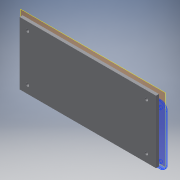
# Autodesk Inventor part: case_bot
Saved by Autodesk Inventor 2019 (Build 230136000, 136)
## iProperties
Created: 2020-04-18
Part Number: case_bot
Material: Generisch
Document SubType Name: Modeling
Designer: marc
Density: 1 g/cm^3
Appearance: Vorgabe
Author: marc
Autodesk Inventor part; units mm, degrees
ref_plane "YZ Plane" through (0, 0, 0) normal (1, 0, 0) x (0, 1, 0)
ref_plane "XZ Plane" through (0, 0, 0) normal (0, 1, 0) x (-1, 0, 0)
ref_plane "XY Plane" through (0, 0, 0) normal (0, 0, 1) x (1, 0, 0)
ref_plane "Arbeitsebene1" through (0, 0, 0) normal (0, 0, 1) x (1, 0, 0)
sketch "Skizze1" plane through (0, 0, 0) normal (0, 0, 1) x (1, 0, 0)
  circle A0 centre (-59.69, 23.2744) radius 1.6 projected
  circle A1 centre (59.69, 23.2744) radius 1.6 projected
  circle A2 centre (59.69, -23.7156) radius 1.6 projected
  circle A3 centre (-59.69, -23.7156) radius 1.6 projected
  circle A4 centre (-59.69, 23.2744) radius 3
  circle A5 centre (59.69, 23.2744) radius 3
  circle A6 centre (59.69, -23.7156) radius 3
  circle A7 centre (-59.69, -23.7156) radius 3
  point P0 (0, 0)
  dimension "d0" = 6
  dimension "d1" = 6
  dimension "d2" = 6
  dimension "d3" = 6
  constraints: 4 centre point, 4 coincident
  measures "d0" diameter of A4
  measures "d1" diameter of A7
  measures "d2" diameter of A5
  measures "d3" diameter of A6
extrude "Extrusion1" add sketch "Skizze1" along normal blind 3
ref_plane "Arbeitsebene2" through (0, 0, 0) normal (0, 0, 1) x (1, 0, 0)
sketch "Skizze2" plane through (0, 0, 0) normal (0, 0, 1) x (1, 0, 0)
  line L0 (-30.04, 15.6244) -> (-27.04, 15.6244)
  line L1 (-27.04, -19.3756) -> (-30.04, -19.3756)
  line L2 (-20.04, 0.6244) -> (-20.04, -4.3756)
  line L3 (-37.04, -4.3756) -> (-37.04, 0.6244)
  line L4 (-1.04, 9.6244) -> (3.96, 9.6244)
  line L5 (3.96, -8.3756) -> (-1.04, -8.3756)
  line L6 (10.96, 0.6244) -> (10.96, -4.3756)
  line L7 (-8.04, -4.3756) -> (-8.04, 0.6244)
  line L8 (40.96, -1.3756) -> (53.96, -1.3756)
  line L9 (53.96, -1.3756) -> (53.96, -4.3756)
  line L10 (53.96, -4.3756) -> (40.96, -4.3756)
  line L11 (40.96, -4.3756) -> (40.96, -1.3756)
  line L12 (-8.04, 0.6244) -> (-1.04, 0.6244)
  line L13 (3.96, 0.6244) -> (10.96, 0.6244)
  line L14 (3.96, 9.6244) -> (3.96, 0.6244)
  line L15 (3.96, -4.3756) -> (3.96, -8.3756)
  line L16 (10.96, -4.3756) -> (3.96, -4.3756)
  line L17 (-1.04, -4.3756) -> (-8.04, -4.3756)
  line L18 (-1.04, -8.3756) -> (-1.04, -4.3756)
  line L19 (-1.04, 0.6244) -> (-1.04, 9.6244)
  line L20 (-37.04, 0.6244) -> (-30.04, 0.6244)
  line L21 (-27.04, 0.6244) -> (-20.04, 0.6244)
  line L22 (-27.04, 15.6244) -> (-27.04, 0.6244)
  line L23 (-27.04, -4.3756) -> (-27.04, -19.3756)
  line L24 (-30.04, -19.3756) -> (-30.04, -4.3756)
  line L25 (-30.04, 0.6244) -> (-30.04, 15.6244)
  line L26 (-20.04, -4.3756) -> (-27.04, -4.3756)
  line L27 (-30.04, -4.3756) -> (-37.04, -4.3756)
  line L28 (-66.04, -24.3506) -> (-66.04, 23.2744) projected
  line L29 (-59.69, 29.6244) -> (59.69, 29.6244) projected
  point P0 (0, 0)
  dimension "d6" = 3
  dimension "d7" = 7
  dimension "d8" = 7
  dimension "d9" = 7
  dimension "d10" = 7
  dimension "d11" = 3
  dimension "d12" = 15
  dimension "d13" = 15
  dimension "d14" = 15
  dimension "d15" = 15
  dimension "d16" = 5
  dimension "d17" = 29
  dimension "d18" = 14
  dimension "d19" = 20
  dimension "d20" = 18
  dimension "d21" = 7
  dimension "d22" = 7
  dimension "d23" = 12
  dimension "d24" = 5
  dimension "d25" = 13
  dimension "d26" = 30
  dimension "d27" = 31
  constraints: 56 end point, 22 parallel, 9 perpendicular, 7 horizontal, 4 horizontal alignment, 2 vertical alignment
  measures "d6" distance of L8.end L9.end
  measures "d7" distance of L21.start L2.start
  measures "d8" distance of L3.end L20.end
  measures "d9" distance of L24.end L3.start
  measures "d10" distance of L2.end L23.start
  measures "d11" distance of L1.start L1.end
  measures "d12" distance of L0.end L21.start
  measures "d13" distance of L23.start L1.start
  measures "d14" distance of L20.end L0.start
  measures "d15" distance of L1.end L24.end
  measures "d16" distance of L2.start L2.end
  measures "d17" distance between parallel lines of L28 L3
  measures "d18" distance between parallel lines of L29 L0
  measures "d19" distance between parallel lines of L29 L4
  measures "d20" distance between parallel lines of L4 L5
  measures "d21" distance of L7.end L12.end
  measures "d22" distance of L13.start L6.start
  measures "d23" distance between parallel lines of L2 L7
  measures "d24" distance of L5.start L5.end
  measures "d25" distance of L8.start L8.end
  measures "d26" distance between parallel lines of L6 L11
  measures "d27" distance between parallel lines of L29 L8
extrude "Extrusion2" add sketch "Skizze2" along normal up to surface (3 mm away)
sketch "Skizze3" plane through (-8.04, 0.6244, 3) normal (0, 0, 1) x (1, 0, 0)
  line L0 (-59.65, 30.65) -> (77.33, 30.65)
  line L1 (77.33, 30.65) -> (77.33, -32.34)
  line L2 (77.33, -32.34) -> (-59.65, -32.34)
  line L3 (-59.65, -32.34) -> (-59.65, 30.65)
  circle A0 centre (67.73, 22.65) radius 1.6 projected
  circle A1 centre (-51.65, 22.65) radius 1.6 projected
  circle A2 centre (-51.65, -24.34) radius 1.6 projected
  circle A3 centre (67.73, -24.34) radius 1.6 projected
  point P0 (8.04, -0.6244)
  dimension "d31" = 8
  dimension "d32" = 8
  dimension "d33" = 8
  dimension "d34" = 8
  constraints: 8 end point, 2 parallel, 1 horizontal, 1 perpendicular
  measures "d31" distance edge to line of A0 L1
  measures "d32" distance from line of L3 A1.centre
  measures "d33" distance from line of L0 A1.centre
  measures "d34" distance from line of L2 A2.centre
extrude "Extrusion3" add sketch "Skizze3" along normal blind 3
fillet "Rundung1" radius 3.75 4 edges at (-62.69, -23.7156, 3) (56.69, -23.7156, 3) (56.69, 23.2744, 3) (-62.69, 23.2744, 3)
sketch "Skizze5" plane through (-8.04, 0.6244, 6) normal (0, 0, 1) x (1, 0, 0)
  circle A0 centre (67.73, 22.65) radius 1.6 projected
  circle A1 centre (67.73, 22.65) radius 6
  circle A2 centre (67.73, -24.34) radius 6
  circle A3 centre (-51.65, 22.65) radius 1.6 projected
  circle A4 centre (-51.65, 22.65) radius 6
  circle A5 centre (-51.65, -24.34) radius 6
  circle A6 centre (-51.65, -24.34) radius 1.6 projected
  circle A7 centre (67.73, -24.34) radius 1.6 projected
  point P0 (8.04, -0.6244)
  dimension "d44" = 12
  dimension "d45" = 12
  dimension "d46" = 12
  dimension "d47" = 12
  constraints: 4 centre point, 2 coincident, 2 concentric
  measures "d44" diameter of A1
  measures "d45" diameter of A2
  measures "d46" diameter of A4
  measures "d47" diameter of A5
extrude "Extrusion5" cut sketch "Skizze5" against normal blind 2
equation "\"d1\" = d0"
equation "\"d2\" = d0"
equation "\"d3\" = d0"
equation "\"d7\" = d8"
equation "\"d9\" = d8"
equation "\"d10\" = d7"
equation "\"d14\" = d12"
equation "\"d15\" = d13"
equation "\"d21\" = d7"
equation "\"d22\" = d7"
equation "\"d32\" = d31"
equation "\"d33\" = d32"
equation "\"d34\" = d33"
equation "\"d45\" = d44"
equation "\"d46\" = d44"
equation "\"d47\" = d46"
